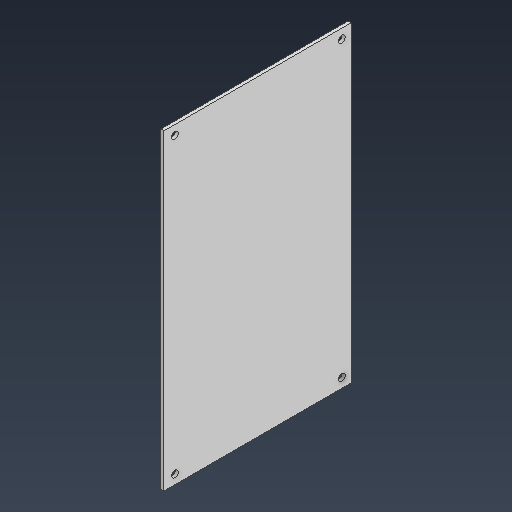
# Autodesk Inventor part: pcb
Saved by Autodesk Inventor 2025.3 (Build 293356000, 356)
## iProperties
Created: 2025-06-10
Part Number: pcb
Material: Generic
Document SubType Name: Modeling
Designer: tolga
Density: 1 g/cm^3
Appearance: Default
Author: tolga
Autodesk Inventor part; units mm, degrees
ref_plane "YZ Plane" through (0, 0, 0) normal (1, 0, 0) x (0, 1, 0)
ref_plane "XZ Plane" through (0, 0, 0) normal (0, 1, 0) x (-1, 0, 0)
ref_plane "XY Plane" through (0, 0, 0) normal (0, 0, 1) x (1, 0, 0)
sketch "Sketch1" plane through (0, 0, 0) normal (1, 0, 0) x (0, 1, 0)
  line L0 (0, 0) -> (100, 0)
  line L1 (100, 0) -> (100, -60)
  line L2 (100, -60) -> (0, -60)
  line L3 (0, -60) -> (0, 0)
  circle A0 centre (97, -57) radius 1.1
  circle A1 centre (97, -3.5) radius 1.1
  circle A2 centre (3, -3.5) radius 1.1
  circle A3 centre (3, -57) radius 1.1
  dimension "d0" = 100
  dimension "d1" = 60
  dimension "d2" = 2.2
  dimension "d3" = 2.2
  dimension "d4" = 3.5
  dimension "d5" = 3
  dimension "d6" = 3
  dimension "d7" = 3
  dimension "d8" = 3
  constraints: 8 end point, 4 centre point, 2 equal radius, 2 parallel, 2 vertical alignment, 1 horizontal, 1 horizontal alignment, 1 perpendicular
  measures "d0" distance of L1.end L2.end
  measures "d1" distance of L0.end L1.end
  measures "d2" diameter of A1
  measures "d3" diameter of A0
  measures "d4" distance from line of L0 A1.centre
  measures "d5" distance from line of L1 A1.centre
  measures "d6" distance from line of L2 A0.centre
  measures "d7" distance from line of L2 A3.centre
  measures "d8" distance from line of L3 A3.centre
extrude "Extrusion1" add sketch "Sketch1" along normal blind 1
equation "\"d3\" = d2"
body "Solid1"
